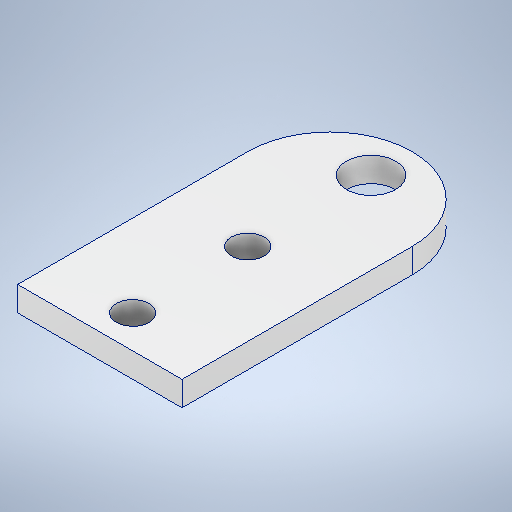
# Autodesk Inventor part: lifter_servo_end
Saved by Autodesk Inventor 2025 (Build 290162000, 162)
## iProperties
Created: 2024-04-25
Part Number: lifter_servo_end
Material: Hliník 6061
Document SubType Name: Modeling
Designer: rader
Density: 2.7 g/cm^3
Appearance: Hliník – plochý
Author: rader
Autodesk Inventor part; units mm, degrees
ref_plane "YZ Plane" through (0, 0, 0) normal (1, 0, 0) x (0, 1, 0)
ref_plane "XZ Plane" through (0, 0, 0) normal (0, 1, 0) x (-1, 0, 0)
ref_plane "XY Plane" through (0, 0, 0) normal (0, 0, 1) x (1, 0, 0)
sketch "Náčrt1" plane through (0, 0, 0) normal (0, 0, 1) x (1, 0, 0)
  line L0 (0, 19) -> (0, 19)
  line L1 (5, 14) -> (5, 0)
  line L2 (0, -19) -> (0, -19)
  line L3 (-5, 0) -> (-5, 14)
  line L4 (-8.4497, 0) -> (8.4497, 0) projected
  line L5 (0, 27.8426) -> (0, -26.8071) projected
  arc A0 (0, 19) -> (-5, 14) centre (0, 14) ccw
  arc A1 (5, 14) -> (0, 19) centre (0, 14) ccw
  line L6 (-5, 0) -> (5, 0)
  point P0 (0, 0)
  point P1 (-5, 19)
  point P2 (5, -19)
  point P3 (5, 19)
  point P4 (0, 19)
  dimension "d2" = 5
  dimension "d12" = 14
  dimension "d13" = 10
  constraints: 10 end point, 6 point on line, 4 point on circle, 4 tangent, 2 centre point, 2 coincident, 2 horizontal, 2 parallel, 1 collinear, 1 concentric, 1 perpendicular, 2 other
  measures "d2" radius of A0
  measures "d12" distance of L1.start L1.end
  measures "d13" distance between parallel lines of L3 L1
extrude "Vysunutí1" add sketch "Náčrt1" along normal mid plane 1.5
sketch "Náčrt2" plane through (0, 0, 0.75) normal (0, 0, 1) x (1, 0, 0)
  line L0 (5, 0) -> (5, 14) projected
  arc A0 (5, 14) -> (-5, 14) centre (0, 14) ccw projected
  line L1 (-5, 14) -> (-5, 0) projected
  line L2 (-5, 0) -> (5, 0) projected
  line L3 (-7, 0) -> (7, 0) projected
  line L4 (0, 25.3) -> (0, -18.8) projected
  point P0 (0, 0)
  point P1 (0, -12.5)
  point P2 (0, 16.5)
  dimension "d23" = 2.5
  constraints: 1 point on line
  measures "d23" distance of A0.centre point (0, 16.5)
hole "Díra1" at (0, -12.5, 0.75) at (0, 16.5, 0.75) direction (0, 0, -1) diameter 3 end through all
sketch "Náčrt3" plane through (0, 0, 0.75) normal (0, 0, 1) x (1, 0, 0)
  line L0 (-5, 14) -> (-5, 0) projected
  line L1 (-5, 0) -> (5, 0) projected
  line L2 (5, 0) -> (5, 14) projected
  arc A0 (5, 14) -> (-5, 14) centre (0, 14) ccw projected
  point P0 (0, 0)
  point P1 (0, 2)
  point P2 (0, 9)
  dimension "d14" = 2
  dimension "d15" = 7
  measures "d14" distance from line of L1 point (0, 2)
  measures "d15" distance of point (0, 2) point (0, 9)
hole "Díra2" at (0, 2, 0.75) at (0, 9, 0.75) direction (0, 0, -1) diameter 2 end through all
